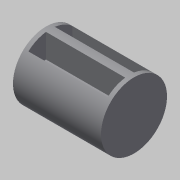
# Autodesk Inventor part: Rounded_beam_body-01
Saved by Autodesk Inventor 2019.3 (Build 233278000, 278)
## iProperties
Created: 2019-02-05
Part Number: Rounded_beam_body-01
Material: Generic
Document SubType Name: Modeling
Designer: Varga Daniel
Density: 1 g/cm^3
Appearance: Default
Beam_body_length: 10,000 mm
Author: Varga Daniel
Autodesk Inventor part; units mm, degrees
ref_plane "YZ Plane" through (0, 0, 0) normal (1, 0, 0) x (0, 1, 0)
ref_plane "XZ Plane" through (0, 0, 0) normal (0, 1, 0) x (-1, 0, 0)
ref_plane "XY Plane" through (0, 0, 0) normal (0, 0, 1) x (1, 0, 0)
derived "Connector_pin_base.ipt"
sketch "Pin_base_sketch" plane through (0, 0, 0) normal (0, 0, 1) x (1, 0, 0)
  line L0 (0, 0) -> (23.0918, 0) construction
  line L1 (0, 0) -> (0, 6.22) construction
  line L2 (0, 3.75) -> (0.55, 3.75)
  line L3 (0.85, 3.45) -> (0.85, 2.4375)
  line L4 (0.85, 2.4375) -> (10.1, 2.4375)
  line L5 (10.1, 2.4375) -> (10.1, 0)
  line L6 (0, 0) -> (0, 3.75)
  line L7 (0, 0) -> (10.1, 0)
  line L8 (9.35, 2.4375) -> (9.35, 2.625)
  line L9 (10.1, 2.4375) -> (10.1, 2.4399)
  arc A0 (10.1, 2.4399) -> (9.9105, 2.7318) centre (9.7805, 2.4399) ccw
  arc A1 (9.9105, 2.7318) -> (9.35, 2.625) centre (9.7071, 2.275) ccw
  line L10 (9.9105, 2.7318) -> (9.9105, -0.0075) construction
  line L11 (8.9584, 2.775) -> (10.3858, 2.775) construction
  arc A2 (0.85, 3.45) -> (0.55, 3.75) centre (0.55, 3.45) ccw
  line L12 (0.85, 2.4375) -> (0.85, 0)
  line L13 (-0.85, 2.4375) -> (-0.85, 0)
  line L14 (-0.85, 3.45) -> (-0.85, 2.4375)
  arc A3 (-0.55, 3.75) -> (-0.85, 3.45) centre (-0.55, 3.45) ccw
  line L15 (0, 3.75) -> (-0.55, 3.75)
  line L16 (0, 0) -> (-23.0918, 0) construction
  line L17 (0, 0) -> (-10.1, 0)
  line L18 (-0.85, 2.4375) -> (-10.1, 2.4375)
  line L19 (-9.35, 2.4375) -> (-9.35, 2.625)
  arc A4 (-9.35, 2.625) -> (-9.9105, 2.7318) centre (-9.7071, 2.275) ccw
  arc A5 (-9.9105, 2.7318) -> (-10.1, 2.4399) centre (-9.7805, 2.4399) ccw
  line L20 (-10.1, 2.4375) -> (-10.1, 2.4399)
  line L21 (-8.9584, 2.775) -> (-10.3858, 2.775) construction
  line L22 (-9.9105, 2.7318) -> (-9.9105, -0.0075) construction
  line L23 (-10.1, 2.4375) -> (-10.1, 0)
  line L24 (9.725, 3.2563) -> (9.725, -1.1868) construction
sketch "Sketch3" plane through (0, 0, 0) normal (1, 0, 0) x (0, 1, 0)
  circle A0 centre (0, 0) radius 3.75
  dimension "d1" = 7.5
  constraints: 1 centre point, 1 coincident
  measures "d1" diameter of A0
extrude "Extrusion1" add sketch "Sketch3" along normal blind 10
sketch "Sketch4" plane through (0, 0, 0) normal (0, 1, 0) x (-1, 0, 0)
  line L0 (0, 0) -> (-73.1618, 0) construction
  line L1 (-10, 3.75) -> (-10, -3.75) construction
  line L2 (-0.5, -2.5) -> (-9.5, -2.5)
  line L3 (-9.5, -2.5) -> (-9.5, -0.5)
  line L4 (-9.5, -0.5) -> (-0.5, -0.5)
  line L5 (-0.5, -0.5) -> (-0.5, -2.5)
  line L6 (0, 0) -> (0, -9.7863) construction
  line L7 (-0.5, 2.5) -> (-9.5, 2.5)
  line L8 (-9.5, 2.5) -> (-9.5, 0.5)
  line L9 (-9.5, 0.5) -> (-0.5, 0.5)
  line L10 (-0.5, 0.5) -> (-0.5, 2.5)
  line L11 (-9.6324, -3.6841) -> (-9.6324, 3.75) construction
  line L12 (0, 3.75) -> (-10, 3.75) construction
  dimension "d4" = 0.5
  dimension "d5" = 2
  dimension "d6" = 9
  dimension "d15" = 0.5
  constraints: 22 end point, 4 symmetric about line, 3 perpendicular, 2 parallel, 1 horizontal, 1 point on line
  measures "d4" distance between parallel lines of L0 L4
  measures "d5" distance between parallel lines of L4 L2
  measures "d6" distance between parallel lines of L3 L5
  measures "d15" distance between parallel lines of L6 L5
extrude "Extrusion2" cut sketch "Sketch4" along normal through all both and the other way through all
extrude "Extrusion3" add sketch "Sketch4" along normal mid plane 2
equation "\"d1\" = Collar_diameter"
equation "\"d2\" = Beam_body_length"
equation "\"Beam_body_length\" = Body_count"
equation "\"Collar_diameter\" = 7.5"
equation "\"Body_count\" = 1"
body "Solid1"
